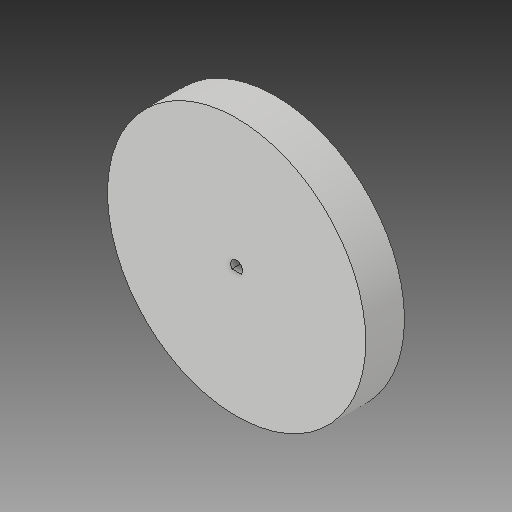
# Autodesk Inventor part: small_wheel
Saved by Autodesk Inventor 2019 (Build 230136000, 136)
## iProperties
Created: 2018-09-24
Part Number: small_wheel
Material: Générique
Document SubType Name: Modeling
Designer: Jérémy
Density: 1 g/cm^3
Appearance: Par défaut
Author: Jérémy
Autodesk Inventor part; units mm, degrees
ref_plane "YZ Plane" through (0, 0, 0) normal (1, 0, 0) x (0, 1, 0)
ref_plane "XZ Plane" through (0, 0, 0) normal (0, 1, 0) x (-1, 0, 0)
ref_plane "XY Plane" through (0, 0, 0) normal (0, 0, 1) x (1, 0, 0)
sketch "Esquisse1" plane through (0, 0, 0) normal (0, 0, 1) x (1, 0, 0)
  arc A0 (1.0724, -0.9466) -> (-1.0724, -0.9466) centre (0, -0.0466) ccw projected
  line L0 (-1.0724, -0.9466) -> (1.0724, -0.9466) projected
  circle A1 centre (0, -0.0466) radius 30
  point P0 (0, 0)
  dimension "d0" = 60
  constraints: 1 centre point, 1 coincident
  measures "d0" diameter of A1
extrude "Extrusion1" add sketch "Esquisse1" against normal blind 9
equation "\"d0\" = d_wheel"
equation "\"d1\" = epaisseur_wheel"
equation "\"epaisseur\" = 6"
equation "\"ecartement\" = 25"
equation "\"dvis\" = 3"
equation "\"largeur\" = 32"
equation "\"L_attache_carte\" = 15"
equation "\"marge_attache_carte\" = 5"
equation "\"L_cubi\" = 81.6"
equation "\"largeur_cubi\" = 81.6"
equation "\"L_moteur\" = 28.3"
equation "\"marge_trou\" = 2"
equation "\"taille_trou\" = 7"
equation "\"H_cubi\" = 81.6"
equation "\"d_wheel\" = 60"
equation "\"epaisseur_wheel\" = 9"
equation "\"H_nez\" = 25"
equation "\"chanfrein\" = 0.5"
equation "\"L_trou_int\" = 1"
equation "\"H_trou_int\" = 0.2"
equation "\"pos_trou_int_1\" = 0.7"
equation "\"pos_trou_int_2\" = 3"
equation "\"epaisseur_metabois\" = 3"
equation "\"L_metabois\" = 8.2"
equation "\"epaisseur_modules\" = 6"
